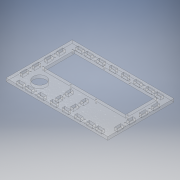
# Autodesk Inventor part: case_top
Saved by Autodesk Inventor 2019 (Build 230136000, 136)
## iProperties
Created: 2019-02-02
Part Number: case_top
Material: Acrylic, Clear
Document SubType Name: Modeling
Designer: suchanek
Density: 1.19 g/cm^3
Appearance: Transparent - Clear
Author: suchanek
Autodesk Inventor part; units mm, degrees
ref_plane "YZ Plane" through (0, 0, 0) normal (1, 0, 0) x (0, 1, 0)
ref_plane "XZ Plane" through (0, 0, 0) normal (0, 1, 0) x (-1, 0, 0)
ref_plane "XY Plane" through (0, 0, 0) normal (0, 0, 1) x (1, 0, 0)
sketch "Sketch1" plane through (0, 0, 0) normal (0, 1, 0) x (-1, 0, 0)
  line L0 (100, 65) -> (-100, 65)
  line L1 (-100, 65) -> (-100, -65)
  line L2 (-100, -65) -> (100, -65)
  line L3 (100, -65) -> (100, 65)
  line L4 (100, 65) -> (-100, -65) construction
  line L5 (-100, 65) -> (100, -65) construction
  line L6 (0, 0) -> (4.5236, 0)
  line L7 (0, 8) -> (0, -20)
  line L8 (0, 0) -> (5.2635, 0)
  line L9 (95.55, -41.85) -> (90.45, -41.85)
  line L10 (90.45, -41.85) -> (90.45, -30.15)
  line L11 (90.45, -30.15) -> (95.55, -30.15)
  line L12 (95.55, -30.15) -> (95.55, -41.85)
  line L13 (95.55, -17.85) -> (90.45, -17.85)
  line L14 (90.45, -17.85) -> (90.45, -6.15)
  line L15 (90.45, -6.15) -> (95.55, -6.15)
  line L16 (95.55, -6.15) -> (95.55, -17.85)
  line L17 (65.85, -55.45) -> (54.15, -55.45)
  line L18 (54.15, -55.45) -> (54.15, -60.55)
  line L19 (54.15, -60.55) -> (65.85, -60.55)
  line L20 (65.85, -60.55) -> (65.85, -55.45)
  line L21 (41.85, -55.45) -> (30.15, -55.45)
  line L22 (30.15, -55.45) -> (30.15, -60.55)
  line L23 (30.15, -60.55) -> (41.85, -60.55)
  line L24 (41.85, -60.55) -> (41.85, -55.45)
  line L25 (17.85, -55.45) -> (6.15, -55.45)
  line L26 (6.15, -55.45) -> (6.15, -60.55)
  line L27 (6.15, -60.55) -> (17.85, -60.55)
  line L28 (17.85, -60.55) -> (17.85, -55.45)
  line L29 (72.15, -60.55) -> (83.85, -60.55)
  line L30 (83.85, -60.55) -> (83.85, -55.45)
  line L31 (83.85, -55.45) -> (72.15, -55.45)
  line L32 (72.15, -55.45) -> (72.15, -60.55)
  line L33 (-95.55, -41.85) -> (-90.45, -41.85)
  line L34 (-90.45, -41.85) -> (-90.45, -30.15)
  line L35 (-90.45, -30.15) -> (-95.55, -30.15)
  line L36 (-95.55, -30.15) -> (-95.55, -41.85)
  line L37 (-95.55, -17.85) -> (-90.45, -17.85)
  line L38 (-90.45, -17.85) -> (-90.45, -6.15)
  line L39 (-90.45, -6.15) -> (-95.55, -6.15)
  line L40 (-95.55, -6.15) -> (-95.55, -17.85)
  line L41 (-65.85, -55.45) -> (-54.15, -55.45)
  line L42 (-54.15, -55.45) -> (-54.15, -60.55)
  line L43 (-54.15, -60.55) -> (-65.85, -60.55)
  line L44 (-65.85, -60.55) -> (-65.85, -55.45)
  line L45 (-41.85, -55.45) -> (-30.15, -55.45)
  line L46 (-30.15, -55.45) -> (-30.15, -60.55)
  line L47 (-30.15, -60.55) -> (-41.85, -60.55)
  line L48 (-41.85, -60.55) -> (-41.85, -55.45)
  line L49 (-17.85, -55.45) -> (-6.15, -55.45)
  line L50 (-6.15, -55.45) -> (-6.15, -60.55)
  line L51 (-6.15, -60.55) -> (-17.85, -60.55)
  line L52 (-17.85, -60.55) -> (-17.85, -55.45)
  line L53 (-72.15, -60.55) -> (-83.85, -60.55)
  line L54 (-83.85, -60.55) -> (-83.85, -55.45)
  line L55 (-83.85, -55.45) -> (-72.15, -55.45)
  line L56 (-72.15, -55.45) -> (-72.15, -60.55)
  line L57 (95.55, 41.85) -> (90.45, 41.85)
  line L58 (90.45, 41.85) -> (90.45, 30.15)
  line L59 (90.45, 30.15) -> (95.55, 30.15)
  line L60 (95.55, 30.15) -> (95.55, 41.85)
  line L61 (95.55, 17.85) -> (90.45, 17.85)
  line L62 (90.45, 17.85) -> (90.45, 6.15)
  line L63 (90.45, 6.15) -> (95.55, 6.15)
  line L64 (95.55, 6.15) -> (95.55, 17.85)
  line L65 (65.85, 55.45) -> (54.15, 55.45)
  line L66 (54.15, 55.45) -> (54.15, 60.55)
  line L67 (54.15, 60.55) -> (65.85, 60.55)
  line L68 (65.85, 60.55) -> (65.85, 55.45)
  line L69 (41.85, 55.45) -> (30.15, 55.45)
  line L70 (30.15, 55.45) -> (30.15, 60.55)
  line L71 (30.15, 60.55) -> (41.85, 60.55)
  line L72 (41.85, 60.55) -> (41.85, 55.45)
  line L73 (17.85, 55.45) -> (6.15, 55.45)
  line L74 (6.15, 55.45) -> (6.15, 60.55)
  line L75 (6.15, 60.55) -> (17.85, 60.55)
  line L76 (17.85, 60.55) -> (17.85, 55.45)
  line L77 (72.15, 60.55) -> (83.85, 60.55)
  line L78 (83.85, 60.55) -> (83.85, 55.45)
  line L79 (83.85, 55.45) -> (72.15, 55.45)
  line L80 (72.15, 55.45) -> (72.15, 60.55)
  line L81 (-90.45, 30.15) -> (-95.55, 30.15)
  line L82 (-95.55, 17.85) -> (-90.45, 17.85)
  line L83 (-90.45, 17.85) -> (-90.45, 6.15)
  line L84 (-90.45, 6.15) -> (-95.55, 6.15)
  line L85 (-95.55, 6.15) -> (-95.55, 17.85)
  line L86 (-95.55, 41.85) -> (-90.45, 41.85)
  line L87 (-95.55, 30.15) -> (-95.55, 41.85)
  line L88 (-90.45, 41.85) -> (-90.45, 30.15)
  line L89 (-83.85, 55.45) -> (-72.15, 55.45)
  line L90 (-83.85, 60.55) -> (-83.85, 55.45)
  line L91 (-72.15, 60.55) -> (-83.85, 60.55)
  line L92 (-72.15, 55.45) -> (-72.15, 60.55)
  line L93 (-65.85, 60.55) -> (-65.85, 55.45)
  line L94 (-54.15, 55.45) -> (-54.15, 60.55)
  line L95 (-54.15, 60.55) -> (-65.85, 60.55)
  line L96 (-65.85, 55.45) -> (-54.15, 55.45)
  line L97 (-6.15, 55.45) -> (-6.15, 60.55)
  line L98 (-17.85, 55.45) -> (-6.15, 55.45)
  line L99 (-6.15, 60.55) -> (-17.85, 60.55)
  line L100 (-17.85, 60.55) -> (-17.85, 55.45)
  line L101 (-30.15, 55.45) -> (-30.15, 60.55)
  line L102 (-41.85, 60.55) -> (-41.85, 55.45)
  line L103 (-30.15, 60.55) -> (-41.85, 60.55)
  line L104 (-41.85, 55.45) -> (-30.15, 55.45)
  line L105 (80, -50) -> (-80, -50)
  line L106 (-80, -50) -> (-80, 10)
  line L107 (-80, 10) -> (80, 10)
  line L108 (80, 10) -> (80, -50)
  circle A0 centre (63.45, 35.45) radius 12.5
  circle A1 centre (83, -48.875) radius 1.125
  circle A2 centre (-25, -53) radius 1.125
  circle A3 centre (-83, -48.875) radius 1.125
  line L109 (0, -20) -> (17.6, -20)
  circle A4 centre (83, 8.875) radius 1.125
  circle A5 centre (-25, 13) radius 1.125
  circle A6 centre (-83, 8.875) radius 1.125
  circle A7 centre (25, -53) radius 1.125
  circle A8 centre (25, 13) radius 1.125
  circle A9 centre (93, 24) radius 1.125
  circle A10 centre (48, 58) radius 1.125
  circle A11 centre (93, -24) radius 1.125
  circle A12 centre (48, -58) radius 1.125
  circle A13 centre (-93, 24) radius 1.125
  circle A14 centre (-48, 58) radius 1.125
  circle A15 centre (-48, -58) radius 1.125
  circle A16 centre (-93, -24) radius 1.125
  line L110 (17.5, 20.75) -> (12.4, 20.75)
  line L111 (12.4, 20.75) -> (12.4, 30.45)
  line L112 (12.4, 30.45) -> (17.5, 30.45)
  line L113 (17.5, 30.45) -> (17.5, 20.75)
  line L114 (-12.4, 20.75) -> (-17.5, 20.75)
  line L115 (-12.4, 30.45) -> (-12.4, 20.75)
  line L116 (-17.5, 30.45) -> (-12.4, 30.45)
  line L117 (-17.5, 20.75) -> (-17.5, 30.45)
  line L118 (17.5, 40.75) -> (12.4, 40.75)
  line L119 (17.5, 50.45) -> (17.5, 40.75)
  line L120 (12.4, 50.45) -> (17.5, 50.45)
  line L121 (12.4, 40.75) -> (12.4, 50.45)
  line L122 (-12.4, 40.75) -> (-17.5, 40.75)
  line L123 (-12.4, 50.45) -> (-12.4, 40.75)
  line L124 (-17.5, 50.45) -> (-12.4, 50.45)
  line L125 (-17.5, 40.75) -> (-17.5, 50.45)
  circle A17 centre (14.95, 35.6) radius 1.125
  circle A18 centre (-14.95, 35.6) radius 1.125
  point P0 (0, 0)
  point P1 (0, 0)
  dimension "d0" = 130
  dimension "d1" = 200
  dimension "d31" = 5.1
  dimension "d32" = 4.45
  dimension "d34" = 6.15
  dimension "d35" = 11.7
  dimension "d36" = 12.3
  dimension "d37" = 11.7
  dimension "d38" = 6.15
  dimension "d39" = 11.7
  dimension "d40" = 12.3
  dimension "d41" = 11.7
  dimension "d42" = 12.3
  dimension "d43" = 11.7
  dimension "d44" = 6.3
  dimension "d45" = 11.7
  dimension "d46" = 5.1
  dimension "d47" = 4.45
  dimension "d58" = 160
  dimension "d59" = 60
  dimension "d60" = 15
  dimension "d61" = 20
  dimension "d66" = 25
  dimension "d67" = 20
  dimension "d78" = 2.25
  dimension "d80" = 3
  dimension "d81" = 3
  dimension "d82" = 3
  dimension "d83" = 25
  dimension "d84" = 2.55
  dimension "d85" = 6.15
  dimension "d86" = 2.55
  dimension "d87" = 6.15
  dimension "d88" = 5.1
  dimension "d89" = 9.7
  dimension "d92" = 29.9
  dimension "d95" = 20
  dimension "d98" = 5
  dimension "d99" = 2.25
  dimension "d100" = 5.15
  dimension "d101" = 2.55
  dimension "d102" = 27
  constraints: 252 end point, 84 symmetric about line, 21 point on line, 19 centre point, 18 parallel, 13 horizontal, 9 perpendicular, 6 midpoint, 5 collinear, 4 equal radius, 2 vertical, 1 horizontal alignment, 1 tangent, 36 other
  measures "d0" distance of L2.end L0.start
  measures "d1" distance of L1.end L2.end
  measures "d31" distance between parallel lines of L14 L16
  measures "d32" distance between parallel lines of L3 L16
  measures "d34" distance between parallel lines of L15 L8
  measures "d35" distance of L15.end L13.start
  measures "d36" distance between parallel lines of L13 L11
  measures "d37" distance of L11.end L9.start
  measures "d38" distance between parallel lines of L26 L7
  measures "d39" distance of L26.end L27.end
  measures "d40" distance between parallel lines of L28 L22
  measures "d41" distance of L21.start L21.end
  measures "d42" distance between parallel lines of L24 L18
  measures "d43" distance of L17.start L17.end
  measures "d44" distance between parallel lines of L20 L32
  measures "d45" distance of L30.end L31.end
  measures "d46" distance of L25.end L26.end
  measures "d47" distance between parallel lines of L2 L27
  measures "d58" distance of L106.end L107.end
  measures "d59" distance of L105.end L106.end
  measures "d60" distance between parallel lines of L2 L105
  measures "d61" distance between parallel lines of L1 L106
  measures "d66" diameter of A0
  measures "d67" distance from line of L104 A0.centre
  measures "d78" diameter of A1
  measures "d80" distance from line of L105 A2.centre
  measures "d81" distance from line of L108 A1.centre
  measures "d82" distance from line of L106 A3.centre
  measures "d83" distance from line of L7 A2.centre
  measures "d84" distance from line of A10.centre L67
  measures "d85" distance from line of A10.centre L66
  measures "d86" distance from line of L58 A9.centre
  measures "d87" distance from line of L59 A9.centre
  measures "d88" distance of L111.end L112.end
  measures "d89" distance of L110.end L111.end
  measures "d92" distance of L110.start L114.start
  measures "d95" distance of L110.start L118.start
  measures "d98" distance between parallel lines of L73 L120
  measures "d99" diameter of A17
  measures "d100" distance from line of L112 A17.centre
  measures "d101" distance from line of L113 A17.centre
  measures "d102" distance from line of L58 A0.centre
extrude "Extrusion3" add sketch "Sketch1" along normal blind 6
body "Solid3"
